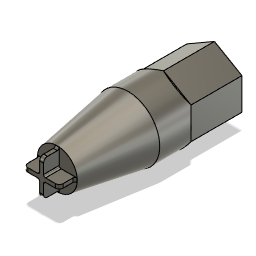
Bit (Autodesk Fusion 360 design; units mm, degrees)
Autodesk Fusion 360 part; units mm, degrees
sketch "Skizze1" plane through (0, 0, 0) normal (0, 0, 1) x (1, 0, 0)
  line L0 (-7, -4.0415) -> (0, -8.0829)
  line L1 (0, -8.0829) -> (7, -4.0415)
  line L2 (7, -4.0415) -> (7, 4.0415)
  line L3 (7, 4.0415) -> (0, 8.0829)
  line L4 (0, 8.0829) -> (-7, 4.0415)
  line L5 (-7, 4.0415) -> (-7, -4.0415)
  dimension "d1" = 14
  constraint vertical L2
  measures "d1" distance of L2 L5
extrude "Extrusion1" add sketch "Skizze1" along normal blind 14
sketch "Skizze2" plane through (0, 0, 14) normal (0, 0, 1) x (1, 0, 0)
  line L0 (-7, 4.0415) -> (-7, -4.0415)
  line L1 (-7, -4.0415) -> (0, -8.0829)
  line L2 (0, -8.0829) -> (7, -4.0415)
  line L3 (7, -4.0415) -> (7, 4.0415)
  line L4 (7, 4.0415) -> (0, 8.0829)
  line L5 (0, 8.0829) -> (-7, 4.0415)
  circle A0 centre (0, 0) radius 8.0829
  constraint coincident A0.centre origin
  constraint coincident L4.end A0
extrude "Extrusion2" add sketch "Skizze2" along normal blind 26
chamfer "Fase1" distance 1.05 angle 45 6 edges at (-3.5, -6.0622, 14) (3.5, -6.0622, 14) (7, 0, 14) (3.5, 6.0622, 14) (-3.5, 6.0622, 14) (-7, 0, 14)
chamfer "Fase2" distance 3 distance2 18 1 edges at (-7.5359, -2.9229, 40) measured on face at (1.2817, -2.0465, 40)
sketch "Skizze3" plane through (0, 0, 40) normal (0, 0, 1) x (1, 0, 0)
  circle A0 centre (0, 0) radius 5.0829
  line L0 (4.5, 0.5) -> (-4.5, 0.5)
  line L1 (-4.5, 0.5) -> (-4.5, -0.5)
  line L2 (-4.5, -0.5) -> (4.5, -0.5)
  line L3 (4.5, -0.5) -> (4.5, 0.5)
  line L4 (4.5, 0.5) -> (-4.5, -0.5) construction
  line L5 (-4.5, 0.5) -> (4.5, -0.5) construction
  line L6 (0.5, 4.5) -> (-0.5, 4.5)
  line L7 (-0.5, 4.5) -> (-0.5, -4.5)
  line L8 (-0.5, -4.5) -> (0.5, -4.5)
  line L9 (0.5, -4.5) -> (0.5, 4.5)
  line L10 (0.5, 4.5) -> (-0.5, -4.5) construction
  line L11 (-0.5, 4.5) -> (0.5, -4.5) construction
  dimension "d9" = 9
  dimension "d10" = 1
  constraint horizontal L0
  constraint perpendicular L0 L1
  constraint parallel L0 L2
  constraint parallel L1 L3
  constraint coincident L4 A0.centre
  constraint coincident L5 A0.centre
  constraint coincident A0.centre origin
  constraint horizontal L6
  constraint perpendicular L6 L7
  constraint parallel L6 L8
  constraint parallel L7 L9
  constraint coincident L10 A0.centre
  constraint coincident L11 A0.centre
  constraint equal L3 L6
  constraint equal L0 L9
  measures "d9" distance of L6.start L8.end
  measures "d10" distance of L6.start L6.end
extrude "Extrusion3" add sketch "Skizze3" along normal blind 4 contours L0 L2 L3 L9 | L0 L2 L7 L9 | L0 L6 L7 L9 | L0 L1 L2 L7 | L2 L7 L8 L9
fillet "Abrundung1" radius 1 4 edges at (0, -4.5, 44) (4.5, 0, 44) (0, 4.5, 44) (-4.5, 0, 44)
fillet "Abrundung2" radius 0.5 4 edges at (-4.5, 0, 40) (0, -4.5, 40) (4.5, 0, 40) (0, 4.5, 40)
fillet "Abrundung3" radius 0.5 4 edges at (0.5, -0.5, 42) (0.5, 0.5, 42) (-0.5, 0.5, 42) (-0.5, -0.5, 42)
sketch "Skizze4" plane through (0, 0, 0) normal (0, 0, -1) x (-1, 0, 0)
  line L0 (7, -4.0415) -> (7, 4.0415)
  line L1 (7, 4.0415) -> (0, 8.0829)
  line L2 (0, 8.0829) -> (-7, 4.0415)
  line L3 (-7, 4.0415) -> (-7, -4.0415)
  line L4 (-7, -4.0415) -> (0, -8.0829)
  line L5 (0, -8.0829) -> (7, -4.0415)
  circle A0 centre (0, 0) radius 5.5
  dimension "d19" = 11
  constraint coincident A0.centre origin
  measures "d19" diameter of A0
extrude "Extrusion4" cut sketch "Skizze4" against normal blind 30 contours A0
chamfer "Fase3" distance 5 distance2 5 1 edges at (5.1278, 1.9889, 30) measured on face at (-5.4727, -0.5476, 20)
fillet "Abrundung4" radius 2 1 edges at (5.1278, -1.9889, 25)
